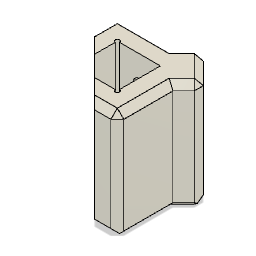
Stereotax_attachment (Autodesk Fusion 360 design; units mm, degrees)
Autodesk Fusion 360 part; units mm, degrees
sketch "Sketch1" plane through (0, 0, 0) normal (0, 1, 0) x (1, 0, 0)
  line L0 (-10, 10) -> (10, 10)
  line L1 (10, 10) -> (10, -10)
  line L2 (10, -10) -> (-10, -10)
  line L3 (-10, -10) -> (-10, 10)
  line L4 (-10, 10) -> (10, -10) construction
  line L5 (10, 10) -> (-10, -10) construction
  line L6 (20, 20) -> (20, -20)
  line L7 (20, -20) -> (-20, -20)
  line L8 (-20, -20) -> (-20, 20)
  line L9 (-20, 20) -> (20, 20)
  dimension "d1" = 20
  dimension "d2" = 20
  dimension "d3" = -10
  constraint perpendicular L0 L1
  constraint parallel L0 L2
  constraint parallel L1 L3
  constraint horizontal L0
  constraint coincident L4 origin
  constraint coincident L5 origin
  measures "d1" distance of L0.end L1.end
  measures "d2" distance of L1.end L2.end
extrude "Extrude1" add sketch "Sketch1" along normal blind 50 makes body 1
sketch "Sketch2" plane through (0, 50, 0) normal (0, 1, 0) x (-1, 0, 0)
  line L0 (-10, 10) -> (10, 10)
  line L1 (10, 10) -> (10, -10)
  line L2 (10, -10) -> (-10, -10)
  line L3 (-10, -10) -> (-10, 10)
  line L4 (20, -20) -> (20, 20)
  line L5 (20, 20) -> (-20, 20)
  line L6 (-20, 20) -> (-20, -20)
  line L7 (-20, -20) -> (20, -20)
ref_plane "WorkPlane1" through (-10, 25, -10) normal (-0.707107, 0, 0.707107) x (0, 1, 0)
ref_plane "WorkPlane2" through (-15.3033, 25, -4.6967) normal (-0.707107, 0, 0.707107) x (0, 1, 0)
split "Split1" by plane through (-15.3033, 25, -4.6967) normal (-0.707107, 0, 0.707107) bodies 1 makes body 2 at (-0.4044, 16.6667, 20)
ref_plane "WorkPlane3" through (20, 25, -20) normal (-0.707107, 0, 0.707107) x (0, 1, 0)
sketch "Sketch3" plane through (20, 25, -20) normal (-0.707107, 0, 0.707107) x (0, 1, 0)
  line L0 (25, -10) -> (-25, -10)
  line L1 (-25, -10) -> (-25, 10)
  line L2 (-25, 10) -> (25, 10)
  line L3 (25, 10) -> (25, -10)
  constraint horizontal L0
  constraint vertical L1
  constraint horizontal L2
  constraint vertical L3
extrude "Extrude2" add sketch "Sketch3" along normal blind 13 and the other way blind 0 bodies 1
sketch "Sketch4" plane through (20, 0, -20) normal (0.707107, 0, -0.707107) x (-0.707107, 0, -0.707107)
  line L0 (-10, 0) -> (10, 0)
  line L1 (10, 0) -> (10, 50)
  line L2 (10, 50) -> (-10, 50)
  line L3 (-10, 50) -> (-10, 0)
  circle A0 centre (0, 25) radius 3.14
  dimension "d13" = 6.28
  measures "d13" diameter of A0
ref_plane "WorkPlane4" through (12.9289, 25, -12.9289) normal (0.707107, 0, -0.707107) x (-0.707107, 0, -0.707107)
sketch "Sketch5" plane through (12.9289, 25, -12.9289) normal (0.707107, 0, -0.707107) x (-0.707107, 0, -0.707107)
  circle A0 centre (0, 0) radius 1.57
  dimension "d15" = 3.14
  constraint coincident A0.centre origin
  measures "d15" diameter of A0
loft "Loft1" cut profiles "Sketch4", "Sketch5" section 1 contours A0 section 2 bodies 1
sketch "Sketch6" plane through (0, 0, -20) normal (0, 0, -1) x (-1, 0, 0)
  line L0 (-5.8579, 50) -> (-5.8579, 0)
  line L1 (-5.8579, 0) -> (20, 0)
  line L2 (20, 0) -> (20, 50)
  line L3 (20, 50) -> (-5.8579, 50)
  line L4 (10, 0) -> (-10, 0)
  line L5 (-10, 0) -> (-10, 50)
  line L6 (-10, 50) -> (10, 50)
  line L7 (10, 50) -> (10, 0)
  line L8 (10, 25) -> (-10, 25) construction
  line L9 (10, 12.5) -> (-10, 12.5) construction
  line L10 (0, 0) -> (0, 25) construction
  circle A0 centre (0, 12.5) radius 2.5
  circle A1 centre (0, 37.5) radius 2.5
  dimension "d16" = 5
  constraint midpoint L7 L8.start
  constraint midpoint L5 L8.end
  constraint coincident L7 L9.start
  constraint coincident L5 L9.end
  constraint perpendicular L5 L9
  constraint coincident L10.start origin
  constraint midpoint L8 L10.end
  constraint midpoint L9 L10
  constraint midpoint L9 A0.centre
  constraint symmetric L8 A0 A1
  measures "d16" diameter of A0
extrude "Extrude3" cut sketch "Sketch6" against normal blind 21 contours A0 | A1 bodies 1
sketch "Sketch7" plane through (0, 0, 0) normal (0, -1, 0) x (1, 0, 0)
  line L0 (12.9289, -27.0711) -> (27.0711, -12.9289)
  line L1 (27.0711, -12.9289) -> (20, -5.8579)
  line L2 (20, -5.8579) -> (20, 20)
  line L3 (20, 20) -> (9.3934, 20)
  line L4 (9.3934, 20) -> (-0.6066, 10)
  line L5 (-0.6066, 10) -> (10, 10)
  line L6 (10, 10) -> (10, -10)
  line L7 (10, -10) -> (-10, -10)
  line L8 (-10, -10) -> (-10, 0.6066)
  line L9 (-10, 0.6066) -> (-20, -9.3934)
  line L10 (-20, -9.3934) -> (-20, -20)
  line L11 (-20, -20) -> (5.8579, -20)
  line L12 (5.8579, -20) -> (12.9289, -27.0711)
  circle A0 centre (-10, -10) radius 1
  circle A1 centre (10, 10) radius 1
  dimension "d21" = 2
  dimension "d22" = 2
  constraint coincident L7.end L8.start
  constraint coincident L5.end L6.start
  measures "d21" diameter of A0
  measures "d22" diameter of A1
extrude "Extrude4" cut sketch "Sketch7" against normal blind 53 contours L7 L8 A0 | L5 L6 A1 picked at (-9.3369, -10.0489) picked at (10, 10.6648) bodies 1
chamfer "Chamfer1" distance 3 angle 45 16 edges at (20, 25, 20) (27.0711, 25, -12.9289) (12.9289, 25, -27.0711) (20, 50, -20) (20, 0, -20) (20, 50, 7.0711) (23.5355, 50, -9.3934) (9.3934, 50, -23.5355) (-7.0711, 50, -20) (-20, 25, -20) (-7.0711, 0, -20) (9.3934, 0, -23.5355) (-20, 0, -14.6967) (14.6967, 0, 20) (-20, 50, -14.6967) (14.6967, 50, 20) on bodies 1
chamfer "Chamfer2" distance 2 angle 45 2 edges at (20, 0, 5.5711) (22.4749, 0, -8.3327) on bodies 1
extrude "Extrude5" cut 1 faces at (13.1588, 25.9211, -12.6991) along direction (-0.707107, 0, 0.707107) blind 17 on bodies 1 bodies 1
hidden bodies 2
equation "d1 = sqUARELENGTH"
equation "d2 = sqUARELENGTH"
equation "d3 = shellthickness"
equation "shellthickness = -10 mm"
equation "sqUARELENGTH = 20 mm"
